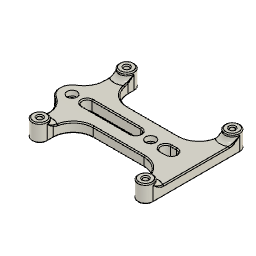
Toolhead Breakout PCB Bracket (Autodesk Fusion 360 design; units mm, degrees)
Autodesk Fusion 360 part; units mm, degrees
sketch "Sketch1" plane through (0, 0, 0) normal (0, 0, 1) x (1, 0, 0)
  line L0 (21.185, 17.41) -> (-21.185, 17.41) construction
  line L1 (-21.185, 17.41) -> (-21.185, -17.41) construction
  line L2 (-21.185, -17.41) -> (21.185, -17.41) construction
  line L3 (21.185, -17.41) -> (21.185, 17.41) construction
  line L4 (21.185, 17.41) -> (-21.185, -17.41) construction
  line L5 (-21.185, 17.41) -> (21.185, -17.41) construction
  circle A0 centre (-21.185, 17.41) radius 0.95
  circle A1 centre (-21.185, -17.41) radius 0.95
  circle A2 centre (21.185, -17.41) radius 0.95
  circle A3 centre (21.185, 17.41) radius 0.95
  circle A4 centre (-21.185, 17.41) radius 3
  circle A5 centre (21.185, 17.41) radius 3
  circle A6 centre (21.185, -17.41) radius 3
  circle A7 centre (-21.185, -17.41) radius 3
  line L6 (0, 0) -> (0, 14.4635) construction
  line L7 (0, 0) -> (27.8853, 0) construction
  circle A8 centre (5.85, 0) radius 1.2
  circle A9 centre (-25.65, 0) radius 1.2
  line L8 (0, 0) -> (-25.65, 0) construction
  line L9 (18.185, 17.41) -> (24.185, 17.41) construction
  line L10 (24.185, 17.41) -> (24.185, -17.41)
  line L11 (24.185, -17.41) -> (18.185, -17.41) construction
  line L12 (18.185, -17.41) -> (18.185, 17.41)
  line L13 (18.185, -7) -> (-18.185, -7)
  line L14 (-18.185, -7) -> (-18.185, 7)
  line L15 (-18.185, 7) -> (18.185, 7)
  line L16 (18.185, 7) -> (18.185, -7)
  line L17 (-18.185, 17.41) -> (-24.185, 17.41)
  line L18 (-24.185, 17.41) -> (-24.185, -17.41)
  line L19 (-24.185, -17.41) -> (-18.185, -17.41)
  line L20 (-18.185, -17.41) -> (-18.185, 17.41)
  circle A10 centre (-25.65, 0) radius 5
  line L21 (-28.433, 4.1539) -> (-24.185, 7)
  line L22 (-18.185, 7) -> (-24.185, 7) construction
  line L23 (-28.433, -4.1539) -> (-24.185, -7)
  dimension "d1" = 42.37
  dimension "d2" = 34.82
  dimension "d3" = 1.9
  dimension "d4" = 6
  dimension "d32" = 5.85
  dimension "d33" = 31.5
  dimension "d34" = 2.4
  dimension "d35" = 14
  dimension "d36" = 10
  constraint horizontal L0
  constraint perpendicular L0 L1
  constraint parallel L0 L2
  constraint parallel L1 L3
  constraint coincident L4 L6.start
  constraint coincident L5 L6.start
  constraint coincident L6.start L7.start
  constraint coincident L0.end L1.start
  constraint coincident L1.end L2.start
  constraint coincident L2.end L3.start
  constraint coincident L0.start L3.end
  constraint equal A0 A3
  constraint equal A0 A1
  constraint equal A0 A2
  constraint concentric A0 A4
  constraint concentric A3 A5
  constraint concentric A2 A6
  constraint concentric A1 A7
  constraint equal A4 A5
  constraint equal A4 A7
  constraint equal A4 A6
  constraint perpendicular L0 L6
  constraint perpendicular L6 L7
  constraint coincident L7 A8.centre
  constraint coincident A9.centre L8.end
  constraint perpendicular L1 L8
  constraint equal A8 A9
  constraint horizontal L9
  constraint vertical L10
  constraint horizontal L11
  constraint vertical L12
  constraint coincident L0 L9.start
  constraint coincident A5 L9.start
  constraint tangent A6 L10
  constraint coincident A6 L10.end
  constraint horizontal L13
  constraint vertical L14
  constraint horizontal L15
  constraint vertical L16
  constraint coincident L12 L13.start
  constraint midpoint L12 L16
  constraint horizontal L17
  constraint vertical L18
  constraint horizontal L19
  constraint vertical L20
  constraint coincident A4 L17.start
  constraint coincident L0 L17.start
  constraint tangent A7 L18
  constraint coincident A7 L18.end
  constraint concentric A9 A10
  constraint coincident L13.end L20
  constraint coincident L18 L21.end
  constraint tangent A10 L21
  constraint coincident A10 L21.start
  constraint perpendicular L18 L22
  constraint symmetric L8 L21.start L23.start
  constraint symmetric L8 L21.end L23.end
  measures "d1" distance of L0.start L0.end
  measures "d2" distance of L0.end L1.end
  measures "d3" diameter of A3
  measures "d4" diameter of A4
  measures "d32" distance of L6.start A8.centre
  measures "d33" distance of A8.centre A9.centre
  measures "d34" diameter of A9
  measures "d35" distance of L13 L15
  measures "d36" diameter of A10
extrude "Extrude1" add sketch "Sketch1" along normal blind 4 contours A0 A4 L17 | A0 A4 L17 | A4 A7 L14 L18 L20 A10 | L12 L13 L14 L15 L16 L20 | L18 A10 L21 | A5 A6 L10 L12 L16 | L18 A10 | L18 A10 | A1 A7 L19 | A1 A7 L19 | A5 | L18 A10 L23 | A6
sketch "Sketch7" plane through (0, 0, 4) normal (0, 0, 1) x (-1, 0, 0)
  circle A0 centre (21.185, 17.41) radius 0.95
  circle A1 centre (21.185, -17.41) radius 0.95
  circle A2 centre (-5.85, 0) radius 1.2
  circle A3 centre (25.65, 0) radius 1.2
  circle A4 centre (-21.185, -17.41) radius 0.95
  circle A5 centre (-21.185, 17.41) radius 0.95
  arc A6 (28.433, -4.1539) -> (28.433, 4.1539) centre (25.65, 0) ccw
  line L0 (28.433, 4.1539) -> (24.185, 7)
  line L1 (24.185, 7) -> (24.185, 17.41)
  arc A7 (24.185, 17.41) -> (18.185, 17.41) centre (21.185, 17.41) ccw
  line L2 (18.185, 17.41) -> (18.185, 7)
  line L3 (18.185, 7) -> (-18.185, 7)
  line L4 (-18.185, 7) -> (-18.185, 17.41)
  arc A8 (-18.185, 17.41) -> (-24.185, 17.41) centre (-21.185, 17.41) ccw
  line L5 (-24.185, 17.41) -> (-24.185, -17.41)
  arc A9 (-24.185, -17.41) -> (-18.185, -17.41) centre (-21.185, -17.41) ccw
  line L6 (-18.185, -17.41) -> (-18.185, -7)
  line L7 (-18.185, -7) -> (18.185, -7)
  line L8 (18.185, -7) -> (18.185, -17.41)
  arc A10 (18.185, -17.41) -> (24.185, -17.41) centre (21.185, -17.41) ccw
  line L9 (24.185, -17.41) -> (24.185, -7)
  line L10 (24.185, -7) -> (28.433, -4.1539)
  circle A11 centre (21.185, -17.41) radius 3
  circle A12 centre (21.185, 17.41) radius 3
  circle A13 centre (-21.185, -17.41) radius 3
  circle A14 centre (-21.185, 17.41) radius 3
  constraint concentric A1 A11
  constraint concentric A0 A12
  constraint concentric A4 A13
  constraint concentric A5 A14
extrude "Extrude7" add sketch "Sketch7" along normal blind 3 contours A10 A11 | A7 A12 | A9 A13 | A8 A14
sketch "Sketch8" plane through (0, 0, 4) normal (0, 0, 1) x (-1, 0, 0)
  arc A0 (24.185, -17.41) -> (18.185, -17.41) centre (21.185, -17.41) ccw
  line L0 (24.185, -17.41) -> (24.185, -7)
  line L1 (24.185, -7) -> (28.433, -4.1539)
  arc A1 (28.433, -4.1539) -> (28.433, 4.1539) centre (25.65, 0) ccw
  line L2 (28.433, 4.1539) -> (24.185, 7)
  line L3 (24.185, 7) -> (24.185, 17.41)
  arc A2 (18.185, 17.41) -> (24.185, 17.41) centre (21.185, 17.41) ccw
  line L4 (18.185, 17.41) -> (18.185, 7)
  line L5 (18.185, 7) -> (-18.185, 7)
  line L6 (-18.185, 7) -> (-18.185, 17.41)
  arc A3 (-24.185, 17.41) -> (-18.185, 17.41) centre (-21.185, 17.41) ccw
  line L7 (-24.185, 17.41) -> (-24.185, -17.41)
  arc A4 (-18.185, -17.41) -> (-24.185, -17.41) centre (-21.185, -17.41) ccw
  line L8 (-18.185, -17.41) -> (-18.185, -7)
  line L9 (-18.185, -7) -> (18.185, -7)
  line L10 (18.185, -7) -> (18.185, -17.41)
  circle A5 centre (-5.85, 0) radius 1.2
  circle A6 centre (25.65, 0) radius 1.2
  circle A7 centre (25.65, 0) radius 2
  circle A8 centre (-5.85, 0) radius 2
  dimension "d39" = 4
  constraint concentric A1 A7
  constraint concentric A5 A8
  constraint equal A7 A8
  measures "d39" diameter of A7
extrude "Extrude8" cut sketch "Sketch8" against normal blind 2 contours A7 | A8
sketch "Sketch9" plane through (0, 0, 4) normal (0, 0, 1) x (-1, 0, 0)
  circle A0 centre (-5.85, 0) radius 2
  circle A1 centre (25.65, 0) radius 2
  arc A2 (24.185, -17.41) -> (18.185, -17.41) centre (21.185, -17.41) ccw
  line L0 (24.185, -17.41) -> (24.185, -7)
  line L1 (24.185, -7) -> (28.433, -4.1539)
  arc A3 (28.433, -4.1539) -> (28.433, 4.1539) centre (25.65, 0) ccw
  line L2 (28.433, 4.1539) -> (24.185, 7)
  line L3 (24.185, 7) -> (24.185, 17.41)
  arc A4 (18.185, 17.41) -> (24.185, 17.41) centre (21.185, 17.41) ccw
  line L4 (18.185, 17.41) -> (18.185, 7)
  line L5 (18.185, 7) -> (-18.185, 7)
  line L6 (-18.185, 7) -> (-18.185, 17.41)
  arc A5 (-24.185, 17.41) -> (-18.185, 17.41) centre (-21.185, 17.41) ccw
  line L7 (-24.185, 17.41) -> (-24.185, -17.41)
  arc A6 (-18.185, -17.41) -> (-24.185, -17.41) centre (-21.185, -17.41) ccw
  line L8 (-18.185, -17.41) -> (-18.185, -7)
  line L9 (-18.185, -7) -> (18.185, -7)
  line L10 (18.185, -7) -> (18.185, -17.41)
  line L11 (19.65, -2) -> (0.15, -2)
  line L12 (0.15, -2) -> (0.15, 2) construction
  line L13 (0.15, 2) -> (19.65, 2)
  line L14 (19.65, 2) -> (19.65, -2) construction
  line L15 (-11.85, -2) -> (-14.185, -2)
  line L16 (-14.185, -2) -> (-14.185, 2) construction
  line L17 (-14.185, 2) -> (-11.85, 2)
  line L18 (-11.85, 2) -> (-11.85, -2) construction
  line L19 (0.15, 0) -> (-11.85, 0) construction
  circle A7 centre (19.65, 0) radius 2
  circle A8 centre (0.15, 0) radius 2
  circle A9 centre (-11.85, 0) radius 2
  circle A10 centre (-14.185, 0) radius 2
  dimension "d42" = 6
  dimension "d43" = 6
  dimension "d44" = 4
  dimension "d45" = 6
  dimension "d46" = 10
  constraint horizontal L11
  constraint vertical L12
  constraint horizontal L13
  constraint vertical L14
  constraint horizontal L15
  constraint vertical L16
  constraint horizontal L17
  constraint vertical L18
  constraint equal L12 L18
  constraint horizontal L19
  constraint coincident origin L19
  constraint midpoint L12 L19.start
  constraint midpoint L18 L19.end
  constraint midpoint L14 A7.centre
  constraint coincident L11.start A7
  constraint coincident L19.start A8.centre
  constraint coincident L11.end A8
  constraint coincident L19.end A9.centre
  constraint coincident L15.start A9
  constraint midpoint L16 A10.centre
  constraint coincident L15.end A10
  measures "d42" distance of A1.centre A7.centre
  measures "d43" distance of A0.centre L19.start
  measures "d44" distance of L11.start L13.end
  measures "d45" distance of A0.centre L19.end
  measures "d46" distance of L7 A10.centre
extrude "Extrude9" cut sketch "Sketch9" against normal through all contours L11 L13 A7 A8 | A7 | A8 | A9 A10 | L15 A9 A10 | A9 A10 | A9 A10 | L17 A9 A10
fillet "Fillet5" radius 8 6 edges at (-18.185, -7, 2) (-18.185, 7, 2) (18.185, 7, 2) (18.185, -7, 2) (-24.185, -7, 2) (-24.185, 7, 2)
fillet "Fillet6" radius 2 4 edges at (-21.185, 14.41, 4) (21.185, 14.41, 4) (-21.185, -14.41, 4) (21.185, -14.41, 4)
fillet "Fillet7" radius 0.4 38 edges at (-24.185, -15.5516, 4.6456) (-24.185, -12.3398, 4) (-25.1273, -7.5029, 4) (-28.0826, -4.3887, 4) (-30.65, 0, 4) (-28.0826, 4.3887, 4) (-25.1273, 7.5029, 4) (-24.185, 12.3398, 4) (-24.185, 15.5516, 4.6456) (-18.185, 16.2532, 5.0973) (-18.1556, 14.3166, 4.1158) (-15.291, 8.8413, 4) (0, 7, 4) (15.291, 8.8413, 4) (18.1505, 14.257, 4.0997) (18.185, 16.2532, 5.0973) (-18.185, -16.2532, 5.0973) (-18.1517, -14.2699, 4.103) (-15.291, -8.8413, 4) (0, -7, 4) (15.291, -8.8413, 4) (18.1457, -14.208, 4.0875) (18.185, -16.2532, 5.0973) (24.185, -15.5516, 4.6456) (24.185, 0, 4) (24.185, 15.5516, 4.6456) (-9.9, 2, 4) (1.85, 0, 4) (-9.9, -2, 4) (-21.65, 0, 4) (13.0175, 2, 4) (16.185, 0, 4) (13.0175, -2, 4) (9.85, 0, 4) (-18.388, 18.4948, 7) (-18.388, -16.3252, 7) (23.982, -16.3252, 7) (23.982, 18.4948, 7)
chamfer "Chamfer3" distance 0.4 angle 45 4 edges at (-20.2993, 17.0665, 7) (-20.2993, -17.7535, 7) (22.0707, -17.7535, 7) (22.0707, 17.0665, 7)
chamfer "Chamfer4" distance 0.4 angle 45 22 edges at (0, -7, 0) (-15.8419, -9.3431, 0) (-18.185, -16.205, 0) (-21.185, -20.41, 0) (-24.185, -14.3398, 0) (-25.1273, -7.5029, 0) (-28.0826, -4.3887, 0) (-30.65, 0, 0) (-28.0826, 4.3887, 0) (-25.1273, 7.5029, 0) (-24.185, 14.3398, 0) (-21.185, 20.41, 0) (-18.185, 16.205, 0) (-15.8419, 9.3431, 0) (0, 7, 0) (15.8419, 9.3431, 0) (18.185, 16.205, 0) (21.185, 20.41, 0) (24.185, 0, 0) (21.185, -20.41, 0) (18.185, -16.205, 0) (15.8419, -9.3431, 0)
